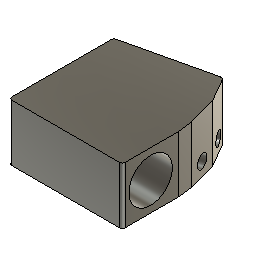
ornithopter (Autodesk Fusion 360 archive; units mm, degrees)
design "spar connector v2.0"
Autodesk Fusion 360 part; units mm, degrees
(part 1 of 2)
sketch "Sketch1" plane through (0, 0, 0) normal (0, 0, 1) x (1, 0, 0)
  line L0 (0, 0) -> (20, 0)
  line L1 (0, 0) -> (20, 0)
  line L2 (20, 0) -> (20, -5)
  line L3 (20, -5) -> (0, -5)
  line L4 (0, -5) -> (0, 0)
  line L5 (20, 0) -> (20, 5)
  line L6 (0, 0) -> (20, 0)
  line L7 (20, 0) -> (20, 5)
  line L8 (20, 5) -> (0, 5)
  line L9 (0, 5) -> (0, 0)
  line L10 (0, 5) -> (18.9894, 10.0882)
  line L11 (0, 5) -> (17.0254, 14.8296)
  line L12 (18.9894, 10.0882) -> (18.3195, 12.5882)
  line L13 (18.3195, 12.5882) -> (15.7313, 17.0711)
  line L14 (0, 5) -> (26.9466, 16.1616)
  line L15 (0, 5) -> (33.8519, 9.4567)
  line L16 (18.9894, 10.0882) -> (19.6593, 7.5882)
  line L17 (19.6593, 7.5882) -> (20, 5)
  line L18 (15.7313, 17.0711) -> (0, 5)
  line L19 (0, 5) -> (0, 13.4392)
  line L20 (0, 13.4392) -> (15.7313, 17.0711)
  dimension "d3" = 20
  dimension "d4" = 5
  dimension "d14" = 15
  dimension "d15" = 15
  dimension "d16" = 7.5
  dimension "d17" = 7.5
  dimension "d37" = 103
  dimension "d38" = 7.5
  constraint coincident L0.start L1.start
  constraint horizontal L0
  constraint horizontal L1
  constraint vertical L2
  constraint horizontal L3
  constraint vertical L4
  constraint perpendicular L1 L5
  constraint equal L2 L5
  constraint horizontal L6
  constraint vertical L7
  constraint horizontal L8
  constraint vertical L9
  constraint perpendicular L10 L12
  constraint perpendicular L11 L13
  constraint coincident L11.end L13
  constraint coincident L12.end L14
  constraint coincident L15 L16.end
  constraint perpendicular L10 L16
  constraint perpendicular L15 L17
  constraint perpendicular L8 L19
  measures "d3" distance of L0.start L0.end
  measures "d4" distance of L1 L3
  measures "d14" angle of L8 L10
  measures "d15" angle of L10 L11
  measures "d16" angle of L10 L14
  measures "d17" angle of L8 L15
  measures "d37" angle of L19 L20
  measures "d38" angle of L11 L18
extrude "Extrude1" add sketch "Sketch1" along normal blind 10
sketch "Sketch2" plane through (20, 0, 0) normal (1, 0, 0) x (0, 1, 0)
  line L0 (-5, 0) -> (5, 0)
  line L1 (5, 10) -> (-5, 10)
  line L2 (-5, 10) -> (-5, 0)
  line L3 (5, 0) -> (5, 10)
  point P0 (0, 5)
hole "Hole1" at (20, 0, 5) direction (-1, 0, 0) diameter 7.65 depth 20 tip angle 118
sketch "Sketch4" plane through (20.2394, 5.4231, 0) normal (0.965926, 0.258819, 0) x (-0.258819, 0.965926, 0)
  line L0 (2.2414, 0) -> (7.4178, 0)
  line L1 (7.4178, 0) -> (7.4178, 10)
  line L2 (7.4178, 10) -> (2.2414, 10)
  line L3 (2.2414, 10) -> (2.2414, 0)
  line L4 (2.2414, 2.35) -> (7.4178, 2.35)
  point P0 (4.8296, 2.35)
  dimension "d18" = 2.35
  constraint coincident L3 L4.start
  constraint coincident L1 L4.end
  constraint perpendicular L1 L4
  constraint midpoint L4 P0
  measures "d18" distance of L0 P0
sketch "Sketch5" plane through (19.1905, 11.0796, 0) normal (0.866025, 0.5, 0) x (-0.5, 0.866025, 0)
  line L0 (1.7419, 0) -> (6.9183, 0)
  line L1 (6.9183, 10) -> (1.7419, 10)
  line L2 (1.7419, 10) -> (1.7419, 0)
  line L3 (1.7419, 2.35) -> (7.3386, 2.35)
  line L4 (6.9183, 0) -> (6.9183, 10)
  point P0 (4.5403, 2.35)
  dimension "d19" = 2.35
  constraint coincident L2 L3.start
  constraint midpoint L3 P0
  measures "d19" distance of L0 L3
sketch "Sketch6" plane through (-2.9457, 12.7591, 0) normal (-0.224951, 0.97437, 0) x (-0.97437, -0.224951, 0)
  line L0 (-19.1683, 0) -> (-3.0232, 0)
  line L1 (-3.0232, 0) -> (-3.0232, 10)
  line L2 (-3.0232, 10) -> (-19.1683, 10)
  line L3 (-19.1683, 10) -> (-19.1683, 0)
  line L4 (-19.1683, 2.85) -> (-3.0232, 2.85)
  point P0 (-8.0232, 2.85)
  dimension "d43" = 2.85
  dimension "d47" = 5
  constraint coincident L3 L4.start
  constraint coincident L1 L4.end
  constraint perpendicular L1 L4
  constraint coincident L4 P0
  measures "d43" distance of L0 L4
  measures "d47" distance of L1 P0
hole "Hole4" at (4.8719, 14.564, 2.85) direction (0.224951, -0.97437, 0) diameter 3.35 depth 10 tip angle 118
hole "Hole2" at (18.9894, 10.0882, 2.35) direction (-0.965926, -0.258819, 0) diameter 2.35 depth 10 tip angle 118
hole "Hole3" at (16.9203, 15.0116, 2.35) direction (-0.866025, -0.5, 0) diameter 2.35 depth 10 tip angle 118
fillet "Fillet1" radius 0.5 1 edges at (15.7313, 17.0711, 5)
fillet "Fillet2" radius 0.5 1 edges at (20, -5, 5)
fillet "Fillet3" radius 0.5 1 edges at (0, 13.4392, 5)
fillet "Fillet4" radius 0.5 1 edges at (0, -5, 5)
mirror "Mirror1" [rolled back] mirror stitch tolerance 0.1
move_body "Move1" [rolled back]
equation "d18 = 5 mm - ( ( 7.65 * 0.5 ) * 1 mm ) + ( 2.35 * 0.5 ) * 1 mm"
equation "d19 = 5 mm - ( 7.65 * 0.5 ) * 1 mm + ( 2.35 * 0.5 ) * 1 mm"
equation "d37 = 180 deg - 77 deg"
equation "d43 = 5 mm - ( 7.65 * 0.5 ) * 1 mm + ( 3.35 * 0.5 ) * 1 mm"

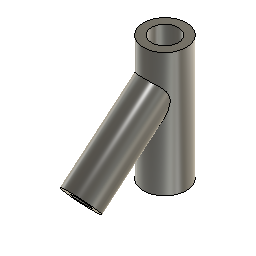
design "spar-to-screw connector"
Autodesk Fusion 360 part; units mm, degrees
sketch "Sketch1" plane through (0, 0, 0) normal (0, 0, 1) x (1, 0, 0)
  circle A0 centre (0, 0) radius 2.632
  circle A1 centre (0, 0) radius 1.632
  dimension "d1" = 3.2639
  dimension "d2" = 1
  constraint coincident A0.centre A1.centre
  constraint concentric A0 A1
  measures "d1" diameter of A1
  measures "d2" distance of A0 A1
extrude "Extrude1" add sketch "Sketch1" along normal blind 15.24 makes body 1
ref_plane "WorkPlane1" through (0, -2.632, 9.1335) normal (0, -1, 0) x (-1, 0, 0)
sketch "Sketch3" plane through (0, -2.632, 9.1335) normal (0, -1, 0) x (1, 0, 0)
  line L0 (-2.6886, 0) -> (2.6498, 0)
  constraint horizontal L0
ref_plane "WorkPlane2" through (-0.0194, -2.632, 9.1335) normal (0, 0.766044, 0.642788) x (1, 0, 0)
sketch "Sketch4" plane through (-0.0194, -2.632, 9.1335) normal (0, 0.766044, 0.642788) x (1, 0, 0)
  circle A0 centre (0, 0) radius 1.175
  circle A1 centre (0, 0) radius 2.175
  line L0 (0, 0) -> (-2.175, 0)
  line L1 (0, 0) -> (2.175, 0)
  dimension "d13" = 2.35
  dimension "d14" = 1
  constraint coincident A0.centre A1.centre
  constraint coincident A1 L0.end
  constraint horizontal L0
  constraint coincident A1 L1.end
  constraint parallel L0 L1
  measures "d13" diameter of A0
  measures "d14" distance of A0 A1
extrude "Extrude4" add sketch "Sketch4" along normal blind 3 separate body contours A0 A1 L0 L1 | A0 A1 L0 L1 makes body 2
extrude "Extrude6" add sketch "Sketch4" against normal blind 10 separate body contours A0 A1 L0 L1 | A0 A1 L0 L1 makes body 3
extrude "Extrude5" cut sketch "Sketch1" along normal blind 16 contours A1 bodies 2
extrude "Extrude7" cut sketch "Sketch1" along normal blind 16 contours A1 bodies 3
combine "Combine1" operation add target body 3 tool bodies 2 1

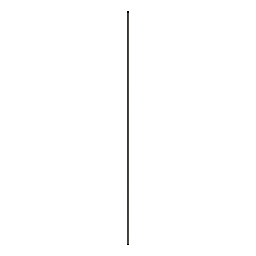
design "small spar medium"
Autodesk Fusion 360 part; units mm, degrees
sketch "Sketch1" plane through (0, 0, 0) normal (0, 0, 1) x (1, 0, 0)
  circle A0 centre (0, 0) radius 1
  dimension "d1" = 2
  constraint coincident A0.centre origin
  measures "d1" diameter of A0
extrude "Extrude1" add sketch "Sketch1" along normal blind 380

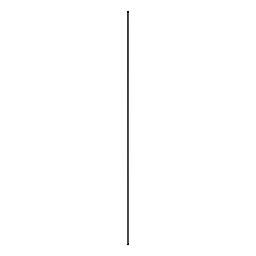
design "small spar long"
Autodesk Fusion 360 part; units mm, degrees
sketch "Sketch1" plane through (0, 0, 0) normal (0, 0, 1) x (1, 0, 0)
  circle A0 centre (0, 0) radius 1
  dimension "d1" = 2
  constraint coincident A0.centre origin
  measures "d1" diameter of A0
extrude "Extrude1" add sketch "Sketch1" along normal blind 423

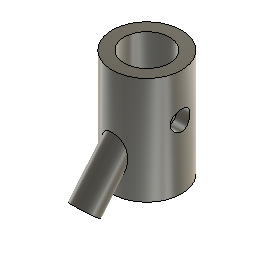
design "spar-to-spar connector large"
Autodesk Fusion 360 part; units mm, degrees
sketch "Sketch1" plane through (0, 0, 0) normal (0, 0, 1) x (1, 0, 0)
  circle A0 centre (0, 0) radius 5.75
  circle A1 centre (0, 0) radius 3.75
  dimension "d1" = 7.5
  dimension "d2" = 2
  constraint coincident A0.centre A1.centre
  constraint concentric A0 A1
  measures "d1" diameter of A1
  measures "d2" distance of A0 A1
extrude "Extrude1" add sketch "Sketch1" along normal blind 17.78 makes body 1
ref_plane "WorkPlane1" through (0, -5.75, 19.9539) normal (0, -1, 0) x (-1, 0, 0)
sketch "Sketch3" plane through (0, -5.75, 9.1335) normal (0, -1, 0) x (1, 0, 0)
  line L0 (-2.6886, 0) -> (2.6498, 0)
  constraint horizontal L0
ref_plane "WorkPlane2" through (-0.0194, -5.75, 9.1335) normal (0, 0.642788, 0.766044) x (1, 0, 0)
sketch "Sketch4" plane through (-0.0194, -3.9203, 7.5982) normal (0, 0.642788, 0.766044) x (1, 0, 0)
  circle A0 centre (0, 0) radius 1.175
  circle A1 centre (0, 0) radius 2.175
  line L0 (0, 0) -> (-2.175, 0)
  line L1 (0, 0) -> (2.175, 0)
  dimension "d13" = 2.35
  dimension "d14" = 1
  constraint coincident A0.centre A1.centre
  constraint coincident A1 L0.end
  constraint horizontal L0
  constraint coincident A1 L1.end
  constraint parallel L0 L1
  measures "d13" diameter of A0
  measures "d14" distance of A0 A1
extrude "Extrude4" add sketch "Sketch4" along normal blind 3 separate body contours A0 A1 L0 L1 | A0 A1 L0 L1 makes body 2
extrude "Extrude6" add sketch "Sketch4" against normal blind 10 separate body contours A0 A1 L0 L1 | A0 A1 L0 L1 makes body 3
extrude "Extrude5" cut sketch "Sketch1" along normal blind 16 contours A1 bodies 2
extrude "Extrude7" cut sketch "Sketch1" along normal blind 16 contours A1 bodies 3
combine "Combine1" operation add target body 3 tool bodies 2 1
ref_plane "WorkPlane3" through (5.75, 0, 13.4902) normal (1, 0, 0) x (0, -1, 0)
sketch "Sketch5" plane through (5.75, 0, 10.5576) normal (1, 0, 0) x (0, 1, 0)
  circle A0 centre (0, 0) radius 1.632
  dimension "d24" = 3.2639
  constraint coincident A0.centre origin
  measures "d24" diameter of A0
extrude "Extrude8" cut sketch "Sketch5" against normal blind 4 bodies 3

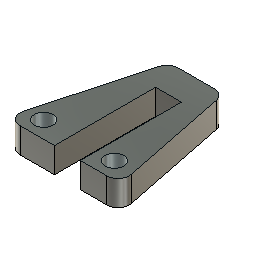
design "screw connector"
Autodesk Fusion 360 part; units mm, degrees
sketch "Sketch1" plane through (0, 0, 0) normal (0, 0, 1) x (1, 0, 0)
  line L0 (15.475, 10) -> (7.4034, 10)
  line L1 (8.375, 10) -> (12.975, 10)
  line L2 (12.975, 10) -> (12.975, 5)
  line L3 (12.975, 5) -> (8.375, 5)
  line L4 (8.375, 5) -> (8.375, 10)
  circle A0 centre (3.4375, -10) radius 1.651
  circle A1 centre (16.05, -10) radius 1.651
  line L5 (5.875, 10) -> (8.375, 10)
  line L6 (12.975, 10) -> (13.8399, 10)
  line L7 (5.4736, 8.5253) -> (0.3022, -10.4747)
  line L8 (2.232, -13) -> (17.693, -13)
  line L9 (19.6531, -10.6025) -> (15.8, 8.3975)
  arc A2 (7.4034, 10) -> (5.4736, 8.5253) centre (7.4034, 8) ccw
  arc A3 (15.8, 8.3975) -> (13.8399, 10) centre (13.8399, 8) ccw
  arc A4 (0.3022, -10.4747) -> (2.232, -13) centre (2.232, -11) ccw
  arc A5 (17.693, -13) -> (19.6531, -10.6025) centre (17.693, -11) ccw
  line L10 (8.375, 5) -> (8.375, -13)
  line L11 (12.975, 5) -> (12.975, -13)
  point P0 (0, 10)
  dimension "d9" = 4.6
  dimension "d11" = 3.302
  dimension "d21" = 20
  dimension "d22" = 20
  dimension "d23" = 2.5
  dimension "d24" = 2.5
  dimension "d25" = 3
  dimension "d26" = 2
  dimension "d27" = 2
  dimension "d28" = 2
  dimension "d29" = 2
  constraint horizontal L0
  constraint horizontal L1
  constraint vertical L2
  constraint horizontal L3
  constraint vertical L4
  constraint coincident L0 L1.start
  constraint equal A0 A1
  constraint coincident P0 L0
  constraint perpendicular L4 L5
  constraint parallel L5 L8
  constraint coincident L5.start L7
  constraint tangent L0 A2
  constraint tangent L7 A2
  constraint coincident L0.start L6
  constraint coincident L0.start L9
  constraint tangent L6 A3
  constraint tangent L9 A3
  constraint tangent L7 A4
  constraint tangent L8 A4
  constraint tangent L8 A5
  constraint tangent L9 A5
  constraint coincident L8 L10.end
  constraint perpendicular L8 L10
  constraint coincident L8 L11.end
  constraint perpendicular L8 L11
  measures "d9" distance of L2 L4
  measures "d11" diameter of A0
  measures "d21" distance of L0 A0.centre
  measures "d22" distance of L0 A1.centre
  measures "d23" distance of L1.start L5.start
  measures "d24" distance of L1.end L0.start
  measures "d25" distance of A0.centre L8
  measures "d26" radius of A2
  measures "d27" radius of A3
  measures "d28" radius of A4
  measures "d29" radius of A5
extrude "Extrude1" add sketch "Sketch1" along normal blind 4.5 contours L0 L2 L6 L8 L9 A3 A5 L11 | L0 L1 L2 L3 L4 | L0 L4 L5 L7 L8 A2 A4 L10
sketch "Sketch2" plane through (0, 0, 4.5) normal (0, 0, 1) x (-1, 0, 0)
  circle A0 centre (-3.4375, 10) radius 1.651
  circle A1 centre (-16.05, 10) radius 1.651
  line L0 (-8.375, -5) -> (-12.975, -5)
  line L1 (-12.975, -5) -> (-12.975, 13)
  line L2 (-12.975, 13) -> (-17.693, 13)
  arc A2 (-17.693, 13) -> (-19.6531, 10.6025) centre (-17.693, 11) ccw
  line L3 (-19.6531, 10.6025) -> (-15.8, -8.3975)
  arc A3 (-15.8, -8.3975) -> (-13.8399, -10) centre (-13.8399, -8) ccw
  line L4 (-13.8399, -10) -> (-7.4034, -10)
  arc A4 (-7.4034, -10) -> (-5.4736, -8.5253) centre (-7.4034, -8) ccw
  line L5 (-5.4736, -8.5253) -> (-0.3022, 10.4747)
  arc A5 (-0.3022, 10.4747) -> (-2.232, 13) centre (-2.232, 11) ccw
  line L6 (-2.232, 13) -> (-8.375, 13)
  line L7 (-8.375, 13) -> (-8.375, -5)

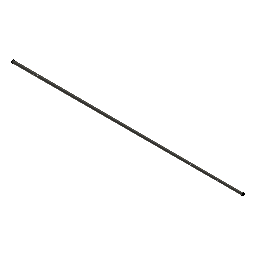
design "large spar"
Autodesk Fusion 360 part; units mm, degrees
sketch "Sketch1" plane through (0, 0, 0) normal (0, 0, 1) x (1, 0, 0)
  line L0 (0, 0) -> (825.5, 0)
  line L1 (825.5, 0) -> (825.5, 7.239)
  line L2 (825.5, 7.239) -> (0, 7.239)
  line L3 (0, 7.239) -> (0, 0)
  line L4 (825.5, 6.4135) -> (825.5, 7.239)
  line L5 (825.5, 1.4097) -> (825.5, 0)
  line L6 (825.5, 0.8255) -> (825.5, 0)
  line L7 (825.5, 6.4135) -> (825.5, 7.239)
  line L8 (825.5, 5.8293) -> (825.5, 6.4135)
  line L9 (825.5, 1.4097) -> (825.5, 0.8255)
  line L10 (0, 6.7183) -> (0, 7.239)
  line L11 (0, 0.5207) -> (0, 0)
  line L12 (0, 6.7183) -> (825.5, 5.8293)
  line L13 (825.5, 1.4097) -> (0, 0.5207)
  line L14 (0, 0) -> (825.5, 0.8255)
  line L15 (825.5, 6.4135) -> (0, 7.239)
  line L16 (0, 3.6195) -> (825.5, 3.6195)
  line L17 (600, 7.239) -> (600, 0)
  point P0 (825.5, 6.4135)
  point P1 (825.5, 5.8293)
  point P2 (825.5, 1.4097)
  point P3 (825.5, 0.8255)
  point P4 (0, 6.7183)
  point P5 (0, 0.5207)
  dimension "d1" = 7.239
  dimension "d2" = 825.5
  dimension "d3" = 5.588
  dimension "d4" = 4.4196
  dimension "d5" = 6.1976
  dimension "d7" = 600
  constraint horizontal L0
  constraint horizontal L2
  constraint vertical L3
  constraint coincident L0.start L3.end
  constraint coincident L1 P0
  constraint coincident L1 P2
  constraint coincident L1 P3
  constraint coincident P0 L4.start
  constraint coincident P2 L5.start
  constraint coincident P3 L6.start
  constraint equal L6 L7
  constraint coincident L1 P1
  constraint coincident P1 L8.start
  constraint equal L8 L9
  constraint coincident L3 P4
  constraint coincident L3 P5
  constraint coincident P4 L10.start
  constraint coincident P5 L11.start
  constraint equal L10 L11
  constraint midpoint L3 L16.start
  constraint midpoint L1 L16.end
  constraint coincident L2 L17.start
  constraint coincident L0 L17.end
  constraint perpendicular L0 L17
  measures "d1" distance of L0 L2
  measures "d2" distance of L1 L3
  measures "d3" distance of P0 P3
  measures "d4" distance of P1 P2
  measures "d5" distance of P4 P5
  measures "d7" distance of L3 L17
revolve "Revolve2" add sketch "Sketch1" angle 360 about axis through (0, 3.6195, 0) along (1, 0, 0) contours L3 L10 L12 L15 L17

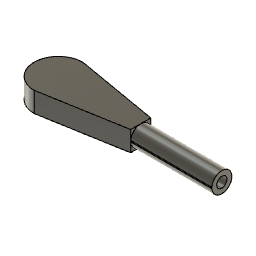
design "servo arm"
Autodesk Fusion 360 part; units mm, degrees
sketch "Sketch1" plane through (0, 0, 0) normal (0, 0, 1) x (1, 0, 0)
  line L0 (0, 0) -> (14.4, 0)
  line L1 (14.4, 0) -> (14.4, 15)
  line L2 (14.4, 15) -> (0, 15)
  line L3 (0, 15) -> (0, 0)
  circle A0 centre (0, 7.5) radius 7.5
  line L4 (0, 15) -> (14.4, 12.5)
  line L5 (0, 0) -> (14.4, 2.5)
  line L6 (14.4, 12.5) -> (25.3509, 10.5988)
  line L7 (14.4, 2.5) -> (25.3509, 4.4012)
  line L8 (25.3509, 4.4012) -> (25.3509, 10.5988)
  dimension "d1" = 15
  dimension "d2" = 14.4
  dimension "d3" = 10
  dimension "d4" = 6.1976
  constraint horizontal L0
  constraint vertical L1
  constraint horizontal L2
  constraint vertical L3
  constraint coincident L0.start L3.end
  constraint midpoint L3 A0.centre
  constraint coincident L2.end A0
  constraint coincident L1 L4.end
  constraint coincident L1 L5.end
  constraint equal L4 L5
  constraint parallel L4 L6
  constraint parallel L5 L7
  constraint coincident L7 L8.start
  constraint coincident L6 L8.end
  constraint perpendicular L2 L8
  constraint coincident L7.end L8.start
  constraint coincident L6.end L8.end
  measures "d1" distance of L0 L2
  measures "d2" distance of L1 L3
  measures "d3" distance of L4.end L5.end
  measures "d4" distance of L7.end L6.end
extrude "Extrude1" add sketch "Sketch1" along normal blind 6.1976 contours L3 A0 | L3 A0 L4 L5 | L1 A0 L4 L5 | L1 L6 L7 L8
sketch "Sketch2" plane through (25.3509, 0, 0) normal (1, 0, 0) x (0, 1, 0)
  line L0 (4.4012, 0) -> (10.5988, 0)
  line L1 (10.5988, 0) -> (10.5988, 6.1976)
  line L2 (10.5988, 6.1976) -> (4.4012, 6.1976)
  line L3 (4.4012, 6.1976) -> (4.4012, 0)
  circle A0 centre (7.4943, 3.0988) radius 3.0988
  circle A1 centre (7.4943, 3.0988) radius 1.5875
  dimension "d7" = 3.175
  constraint tangent L2 A0
  constraint tangent L0 A0
  constraint concentric A0 A1
  measures "d7" diameter of A1
extrude "Extrude2" add sketch "Sketch2" along normal blind 25 contours L3 A0 picked at (7.6808, 0.5158)

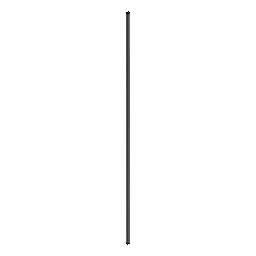
design "medium spar"
Autodesk Fusion 360 part; units mm, degrees
sketch "Sketch1" plane through (0, 0, 0) normal (0, 0, 1) x (1, 0, 0)
  circle A0 centre (0, 0) radius 1.5
  dimension "d1" = 3
  constraint coincident A0.centre origin
  measures "d1" diameter of A0
extrude "Extrude1" add sketch "Sketch1" along normal blind 240

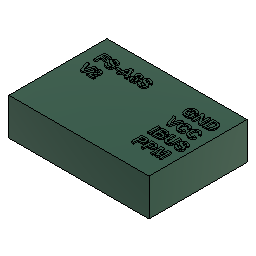
design "reciever"
Autodesk Fusion 360 part; units mm, degrees
sketch "Sketch1" plane through (0, 0, 0) normal (0, 0, 1) x (1, 0, 0)
  line L0 (0, 0) -> (20, 0)
  line L1 (20, 0) -> (20, 14)
  line L2 (20, 14) -> (0, 14)
  line L3 (0, 14) -> (0, 0)
  dimension "d1" = 20
  dimension "d2" = 14
  constraint horizontal L0
  constraint vertical L1
  constraint horizontal L2
  constraint vertical L3
  constraint coincident L0.start L3.end
  measures "d1" distance of L1 L3
  measures "d2" distance of L0 L2
extrude "Extrude1" add sketch "Sketch1" along normal blind 5.3
sketch "Sketch2" plane through (0, 0, 5.3) normal (0, 0, 1) x (-1, 0, 0)
  line L0 (0, -14) -> (0, 0)
  line L1 (0, 0) -> (-20, 0)
  line L2 (-20, 0) -> (-20, -14)
  line L3 (-20, -14) -> (0, -14)
  line L4 (-1.6357, -6.6523) -> (-11.9926, -6.6523) construction
  line L5 (-11.9926, -6.6523) -> (-11.9926, -11.8308) construction
  line L6 (-11.9926, -11.8308) -> (-1.6357, -11.8308) construction
  line L7 (-1.6357, -11.8308) -> (-1.6357, -6.6523) construction
  line L8 (-14.4693, -2.7122) -> (-20, -2.7122) construction
  line L9 (-20, -2.7122) -> (-20, -11.3805) construction
  line L10 (-20, -11.3805) -> (-14.4693, -11.3805) construction
  line L11 (-14.4693, -11.3805) -> (-14.4693, -2.7122) construction
  text T0 "FS-A8S\nV2" font "Arial" height 1.5 bold align left top in box 10.3569 x 5.1784 at (-1.6357, -6.6523) x (-1, 0) y (0, -1) spacing 1 kerned
  text T1 "GND\nVCC\nIBUS\nPPM" font "Arial" height 1.5 bold align left top in box 5.5307 x 8.6683 at (-14.4693, -2.7122) x (-1, 0) y (0, -1) spacing 1 kerned
  constraint coincident L2
emboss "Emboss1" depth 0.2 profiles "Sketch2" section 1 text T1 T0 onto face at (6.6667, 9.3333, 5.3)

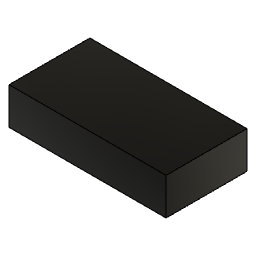
design "battery"
Autodesk Fusion 360 part; units mm, degrees
sketch "Sketch1" plane through (0, 0, 0) normal (0, 0, 1) x (1, 0, 0)
  line L0 (0, 0) -> (68, 0)
  line L1 (68, 0) -> (68, 35)
  line L2 (68, 35) -> (0, 35)
  line L3 (0, 35) -> (0, 0)
  dimension "d1" = 68
  dimension "d2" = 35
  constraint horizontal L0
  constraint vertical L1
  constraint horizontal L2
  constraint vertical L3
  constraint coincident L0.start L3.end
  measures "d1" distance of L1 L3
  measures "d2" distance of L0 L2
extrude "Extrude1" add sketch "Sketch1" along normal blind 16

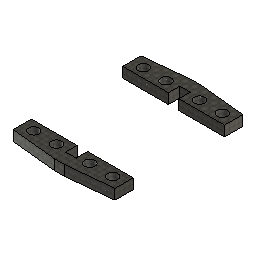
design "servo mount"
Autodesk Fusion 360 part; units mm, degrees
sketch "Sketch1" plane through (0, 0, 0) normal (0, 0, 1) x (1, 0, 0)
  line L0 (0, 0) -> (44.6, 0)
  line L1 (44.6, 0) -> (44.6, 60)
  line L2 (44.6, 60) -> (0, 60)
  line L3 (0, 60) -> (0, 0)
  line L4 (20, 0) -> (36.7004, 0)
  line L5 (0, 0) -> (44.6, 0)
  line L6 (44.6, 0) -> (44.6, 10)
  line L7 (44.6, 10) -> (0, 10)
  line L8 (0, 10) -> (0, 0)
  line L9 (44.6, 60) -> (0, 60)
  line L10 (0, 60) -> (0, 50)
  line L11 (0, 50) -> (44.6, 50)
  line L12 (44.6, 50) -> (44.6, 60)
  line L13 (24.6, 0) -> (44.6, 2)
  line L14 (0, 2) -> (20, 0)
  line L15 (0, 58) -> (20, 60)
  line L16 (24.6, 60) -> (44.6, 58)
  line L17 (20, 50) -> (24.6, 50)
  line L18 (24.6, 50) -> (24.6, 60)
  line L19 (24.6, 60) -> (20, 60)
  line L20 (20, 60) -> (20, 50)
  line L21 (20, 55) -> (24.6, 55)
  line L22 (24.6, 55) -> (24.6, 50)
  line L23 (24.6, 50) -> (20, 50)
  line L24 (20, 50) -> (20, 55)
  line L25 (20, 0) -> (24.6, 0)
  line L26 (24.6, 0) -> (24.6, 10)
  line L27 (24.6, 10) -> (20, 10)
  line L28 (20, 10) -> (20, 0)
  line L29 (20, 10) -> (24.6, 10)
  line L30 (24.6, 10) -> (24.6, 5)
  line L31 (24.6, 5) -> (20, 5)
  line L32 (20, 5) -> (20, 10)
  dimension "d2" = 60
  dimension "d17" = 10
  dimension "d18" = 10
  dimension "d37" = 2
  dimension "d43" = 20
  dimension "d44" = 2
  dimension "d45" = 20
  dimension "d46" = 20
  dimension "d47" = 20
  dimension "d48" = 2
  dimension "d49" = 2
  dimension "d59" = 5
  dimension "d60" = 5
  dimension "d61" = 4.6
  dimension "d62" = 4.6
  constraint horizontal L0
  constraint vertical L1
  constraint horizontal L2
  constraint vertical L3
  constraint coincident L0.start L3.end
  constraint horizontal L4
  constraint coincident L0 L4.start
  constraint horizontal L5
  constraint vertical L6
  constraint horizontal L7
  constraint vertical L8
  constraint coincident L1 L6.end
  constraint horizontal L9
  constraint vertical L10
  constraint horizontal L11
  constraint vertical L12
  constraint coincident L3 L10.end
  constraint coincident L1 L13.end
  constraint coincident L0 L13.start
  constraint coincident L8 L14.start
  constraint coincident L3 L15.start
  constraint coincident L2 L15.end
  constraint coincident L2 L16.start
  constraint coincident L1 L16.end
  constraint horizontal L17
  constraint vertical L18
  constraint horizontal L19
  constraint vertical L20
  constraint coincident L11 L17.start
  constraint horizontal L21
  constraint vertical L22
  constraint horizontal L23
  constraint vertical L24
  constraint coincident L20 L21.start
  constraint horizontal L25
  constraint vertical L26
  constraint horizontal L27
  constraint vertical L28
  constraint coincident L7 L26.end
  constraint horizontal L29
  constraint vertical L30
  constraint horizontal L31
  constraint vertical L32
  constraint coincident L26 L30.end
  constraint coincident L4.start L14.end
  measures "d2" distance of L0 L2
  measures "d17" distance of L5 L7
  measures "d18" distance of L2 L11
  measures "d37" distance of L5 L13.end
  measures "d43" distance of L1 L13.start
  measures "d44" distance of L0.start L14.start
  measures "d45" distance of L0.start L4.start
  measures "d46" distance of L3 L15.end
  measures "d47" distance of L1 L16.start
  measures "d48" distance of L1.end L16.end
  measures "d49" distance of L2.end L15.start
  measures "d59" distance of L17 L21
  measures "d60" distance of L7 L31
  measures "d61" distance of L26 L28
  measures "d62" distance of L22 L24
extrude "Extrude4" add sketch "Sketch1" along normal blind 4.5 contours L0 L4 L5 L25 L26 L28 L31 | L3 L7 L8 L14 L28 L32 | L1 L6 L7 L13 L26 L30 | L3 L10 L11 L15 L20 L24 | L1 L11 L12 L16 L18 L22 | L2 L9 L18 L19 L20 L21 makes body 1 at (6.6667, 54.3333, 0) makes body 2 at (6.6667, 5.6667, 0)
sketch "Sketch3" plane through (0, 0, 4.5) normal (0, 0, 1) x (-1, 0, 0)
  line L0 (-44.6, -50) -> (-44.6, -58)
  line L1 (0, -58) -> (0, -50)
  line L2 (0, -50) -> (-20, -50)
  line L3 (0, -54) -> (-44.6, -54)
  line L4 (-24.6, -60) -> (-20, -60)
  line L5 (-44.6, -58) -> (-24.6, -60)
  line L6 (-20, -60) -> (0, -58)
  line L7 (-20, -50) -> (-20, -55)
  line L8 (-20, -55) -> (-24.6, -55)
  line L9 (-24.6, -55) -> (-24.6, -50)
  line L10 (-24.6, -50) -> (-44.6, -50)
  point P0 (-5, -54)
  point P1 (-15, -54)
  point P2 (-39.6, -54)
  point P3 (-29.6, -54)
  dimension "d24" = 5
  dimension "d25" = 10
  dimension "d26" = 5
  dimension "d27" = 10
  dimension "d50" = 6
  constraint coincident P0 L3
  constraint coincident P1 L3
  constraint coincident P3 L3
  constraint coincident P2 L3
  constraint coincident L0 L3.end
  measures "d24" distance of L1 P0
  measures "d25" distance of P0 P1
  measures "d26" distance of P2 L3.end
  measures "d27" distance of P2 P3
  measures "d50" distance of L3 L4
hole "Hole1" at (5, 54, 4.5) at (15, 54, 4.5) at (29.6, 54, 4.5) at (39.6, 54, 4.5) direction (0, 0, -1) diameter 4.5 depth 20 tip angle 118 bodies 1
sketch "Sketch4" plane through (0, 0, 4.5) normal (0, 0, 1) x (-1, 0, 0)
  line L0 (0, -10) -> (0, -2)
  line L1 (-44.6, -2) -> (-44.6, -10)
  line L2 (-20, -10) -> (0, -10)
  line L3 (0, -6) -> (-44.6, -6)
  line L4 (-24.6, 0) -> (-44.6, -2)
  line L5 (-20, 0) -> (-24.6, 0)
  line L6 (0, -2) -> (-20, 0)
  line L7 (-20, -5) -> (-20, -10)
  line L8 (-44.6, -10) -> (-24.6, -10)
  line L9 (-24.6, -10) -> (-24.6, -5)
  line L10 (-24.6, -5) -> (-20, -5)
  point P0 (-5, -6)
  point P1 (-15, -6)
  point P2 (-29.6, -6)
  point P3 (-39.6, -6)
  dimension "d28" = 5
  dimension "d29" = 10
  dimension "d30" = 5
  dimension "d31" = 10
  dimension "d40" = 6
  constraint coincident L3 P0
  constraint coincident L3 P1
  constraint coincident L3 P2
  constraint coincident L3 P3
  constraint coincident L1 L3.end
  measures "d28" distance of L0 P0
  measures "d29" distance of P0 P1
  measures "d30" distance of L3.end P3
  measures "d31" distance of P2 P3
  measures "d40" distance of L3 L4.start
hole "Hole2" at (5, 6, 4.5) at (15, 6, 4.5) at (29.6, 6, 4.5) at (39.6, 6, 4.5) direction (0, 0, -1) diameter 4.5 depth 20 tip angle 118 bodies 2

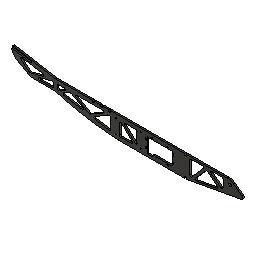
design "frame v2.0"
Autodesk Fusion 360 part; units mm, degrees
sketch "Sketch2" plane through (0, 0, 0) normal (0, 1, 0) x (1, 0, 0)
  line L0 (0, 0) -> (650, 0)
  line L1 (650, 0) -> (650, -200)
  line L2 (650, -200) -> (0, -200)
  line L3 (0, -200) -> (0, 0)
  line L4 (0, -81.4313) -> (0, -60)
  line L5 (54, -30) -> (0, -60)
  line L6 (54, -30) -> (121.5, -29.9038)
  line L7 (121.5, -29.9038) -> (121.4776, -14.1987)
  line L8 (121.5, -29.9038) -> (121.5429, -60)
  line L9 (121.5429, -60) -> (610.012, -60)
  line L10 (610.012, -60) -> (650, -30)
  line L11 (650, -30) -> (486, 0)
  line L12 (486, 0) -> (297, 0)
  line L13 (297, 0) -> (121.4776, -14.1987)
  line L14 (0, -81.4313) -> (121.5429, -60)
  point P0 (650, -679.9029)
  point P1 (201.3394, 90.956)
  point P2 (486, 0)
  point P3 (-7419.8633, 0)
  point P4 (0, -60)
  point P5 (0, -81.4313)
  point P6 (121.5429, -60)
  point P7 (54, -30)
  point P8 (121.5, -29.9038)
  point P9 (121.4776, -14.1987)
  point P10 (297, 0)
  point P11 (650, -30)
  point P12 (610.012, -60)
  dimension "d5" = 650
  dimension "d6" = 200
  dimension "d30" = 60
  dimension "d32" = 30
  dimension "d33" = 54
  dimension "d34" = 121.5
  dimension "d36" = 60
  dimension "d37" = 297
  dimension "d38" = 486
  dimension "d39" = 30
  dimension "d40" = 60
  dimension "d80" = 170
  constraint horizontal L0
  constraint vertical L1
  constraint horizontal L2
  constraint vertical L3
  constraint coincident L0.start L3.end
  constraint coincident L1 P0
  constraint coincident L0 P2
  constraint coincident L0 P3
  constraint coincident L3 P4
  constraint coincident L3 P5
  constraint coincident L0 P10
  constraint coincident L1 P11
  constraint coincident P5 L4.start
  constraint coincident P4 L4.end
  constraint coincident P7 L5.start
  constraint coincident P8 L6.end
  constraint coincident P9 L7.end
  constraint perpendicular L6 L7
  constraint coincident P6 L8.end
  constraint parallel L7 L8
  constraint coincident P12 L9.end
  constraint coincident P11 L10.end
  constraint coincident P2 L11.end
  constraint coincident P10 L12.end
  measures "d5" distance of L1 L3
  measures "d6" distance of L0 L2
  measures "d30" distance of L0 P4
  measures "d32" distance of L0 P7
  measures "d33" distance of L3 P7
  measures "d34" distance of L3 P8
  measures "d36" distance of L0 P6
  measures "d37" distance of L0.start P10
  measures "d38" distance of L3 P2
  measures "d39" distance of L0 P11
  measures "d40" distance of L0 P12
  measures "d80" angle of L9 L14
extrude "Extrude3" add sketch "Sketch2" along normal blind 4.5 contours L0 L7 L8 L9 L10 L11 L12 L13 | L3 L4 L5 L6 L8 L14
sketch "Sketch4" plane through (0, 0, 0) normal (0, -1, 0) x (1, 0, 0)
  line L0 (0, 81.4313) -> (0, 60)
  line L1 (0, 60) -> (54, 30)
  line L2 (54, 30) -> (121.5, 29.9038)
  line L3 (121.5, 29.9038) -> (121.4776, 14.1987)
  line L4 (121.4776, 14.1987) -> (297, 0)
  line L5 (297, 0) -> (486, 0)
  line L6 (486, 0) -> (650, 30)
  line L7 (650, 30) -> (610.012, 60)
  line L8 (610.012, 60) -> (121.5429, 60)
  line L9 (486, 0) -> (481.4, 0)
  line L10 (481.4, 0) -> (481.4, 60)
  line L11 (481.4, 60) -> (486, 60)
  line L12 (486, 60) -> (486, 0)
  line L13 (481.4, 60) -> (486, 60)
  line L14 (486, 60) -> (486, 55)
  line L15 (486, 55) -> (481.4, 55)
  line L16 (481.4, 55) -> (481.4, 60)
  line L17 (481.4, 0) -> (486, 0)
  line L18 (486, 0) -> (486, 5)
  line L19 (486, 5) -> (481.4, 5)
  line L20 (481.4, 5) -> (481.4, 0)
  line L21 (121.5429, 60) -> (0, 81.4313)
  dimension "d57" = 4.6
  dimension "d58" = 5
  constraint horizontal L9
  constraint vertical L10
  constraint horizontal L11
  constraint vertical L12
  constraint coincident L8 L10.end
  constraint coincident L5.end L6.start
  constraint horizontal L13
  constraint vertical L14
  constraint horizontal L15
  constraint vertical L16
  constraint coincident L12 L14.end
  constraint horizontal L17
  constraint vertical L18
  constraint horizontal L19
  constraint vertical L20
  constraint equal L16 L20
  measures "d57" distance of L10 L12
  measures "d58" distance of L5 L19.end
extrude "Extrude5" cut sketch "Sketch4" against normal blind 5 contours L8 L10 L11 L12 L13 L14 L15 L16 | L5 L9 L10 L12 L17 L18 L19 L20
fillet "Fillet16" radius 730 1 edges at (121.4776, 2.25, 14.1987)
fillet "Fillet17" radius 5 1 edges at (650, 2.25, 30)
fillet "Fillet18" radius 30 1 edges at (610.012, 2.25, 60)
fillet "Fillet19" radius 30 1 edges at (54, 2.25, 30)
fillet "Fillet20" radius 30 1 edges at (0, 2.25, 60)
fillet "Fillet22" radius 5 1 edges at (0, 2.25, 81.4313)
sketch "Sketch21" plane through (0, 0, 0) normal (0, -1, 0) x (1, 0, 0)
  arc A0 (5.9649, 80.3795) -> (0.116, 75.0161) centre (5.0967, 75.4555) ccw
  arc A1 (0.116, 75.0161) -> (15.4307, 51.4274) centre (30, 77.6521) ccw
  line L0 (15.4307, 51.4274) -> (47.2244, 33.7642)
  arc A2 (47.2244, 33.7642) -> (61.751, 29.989) centre (61.7937, 59.9889) ccw
  line L1 (61.751, 29.989) -> (121.5, 29.9038)
  arc A3 (121.5, 29.9038) -> (270.1218, 2.1743) centre (328.9822, 729.7974) ccw
  line L2 (270.1218, 2.1743) -> (297, 0)
  line L3 (297, 0) -> (481.4, 0)
  line L4 (481.4, 0) -> (481.4, 5)
  line L5 (481.4, 5) -> (486, 5)
  line L6 (486, 5) -> (486, 0)
  line L7 (486, 0) -> (638.7541, 27.9428)
  arc A4 (638.7541, 27.9428) -> (640.855, 36.8608) centre (637.8544, 32.8612) ccw
  line L8 (640.855, 36.8608) -> (618.013, 53.9974)
  arc A5 (618.013, 53.9974) -> (600.0096, 60) centre (600.0096, 30) ccw
  line L9 (600.0096, 60) -> (486, 60)
  line L10 (486, 60) -> (486, 55)
  line L11 (486, 55) -> (481.4, 55)
  line L12 (481.4, 55) -> (481.4, 60)
  line L13 (481.4, 60) -> (121.5429, 60)
  line L14 (121.5429, 60) -> (5.9649, 80.3795)
  line L15 (121.5429, 60) -> (5.9649, 80.3795)
  line L16 (5.9649, 80.3795) -> (4.6452, 72.895)
  line L17 (4.6452, 72.895) -> (120.2232, 52.5155)
  line L18 (120.2232, 52.5155) -> (121.5429, 60)
  line L19 (121.022, 57.0456) -> (5.444, 77.4251)
  line L20 (4.6452, 72.895) -> (5.444, 77.4251)
  line L21 (5.444, 77.4251) -> (-21.9849, 82.2615)
  line L22 (-21.9849, 82.2615) -> (-22.7836, 77.7314)
  line L23 (-22.7836, 77.7314) -> (4.6452, 72.895)
  line L24 (55.444, 68.6087) -> (54.6452, 64.0786)
  dimension "d201" = 50
  dimension "d213" = 4.6
  dimension "d215" = 3
  constraint perpendicular L15 L16
  constraint parallel L15 L17
  constraint parallel L16 L18
  constraint coincident A0.start L14.end
  constraint tangent A0 L15
  constraint coincident L13.end L14.start
  constraint perpendicular L20 L21
  constraint parallel L20 L22
  constraint parallel L21 L23
  constraint coincident L19 L24.start
  constraint coincident L17 L24.end
  constraint perpendicular L17 L24
  constraint parallel L19 L21
  constraint parallel L15 L19
  measures "d201" horizontal distance of L16.end L24.end
  measures "d213" distance of L21 L23
  measures "d215" distance of L15 L19
extrude "Extrude13" cut sketch "Sketch21" against normal blind 10 contours A0 A1 L16 L20 L21 L23 | L16 L17 L19 L20 L24
sketch "Sketch7" plane through (0, 0, 0) normal (0, -1, 0) x (1, 0, 0)
  arc A0 (0.2658, 73.6672) -> (15.4307, 51.4274) centre (30, 77.6521) ccw
  line L0 (15.4307, 51.4274) -> (47.2244, 33.7642)
  arc A1 (47.2244, 33.7642) -> (61.751, 29.989) centre (61.7937, 59.9889) ccw
  line L1 (61.751, 29.989) -> (121.5, 29.9038)
  arc A2 (121.5, 29.9038) -> (270.1218, 2.1743) centre (328.9822, 729.7974) ccw
  line L2 (270.1218, 2.1743) -> (297, 0)
  line L3 (297, 0) -> (481.4, 0)
  line L4 (481.4, 0) -> (481.4, 5)
  line L5 (481.4, 5) -> (486, 5)
  line L6 (486, 5) -> (486, 0)
  line L7 (486, 0) -> (638.7541, 27.9428)
  arc A3 (638.7541, 27.9428) -> (640.855, 36.8608) centre (637.8544, 32.8612) ccw
  line L8 (640.855, 36.8608) -> (618.013, 53.9974)
  arc A4 (618.013, 53.9974) -> (600.0096, 60) centre (600.0096, 30) ccw
  line L9 (600.0096, 60) -> (486, 60)
  line L10 (486, 60) -> (486, 55)
  line L11 (486, 55) -> (481.4, 55)
  line L12 (481.4, 55) -> (481.4, 60)
  line L13 (378.4, 48) -> (445.4, 48)
  line L14 (446.4, 48) -> (446.4, 12)
  line L15 (445.4, 12) -> (378.4, 12)
  line L16 (377.4, 12) -> (377.4, 47)
  line L17 (377.4, 48) -> (377.4, 60)
  line L18 (377.4, 12) -> (377.4, 0)
  line L19 (481.4, 60) -> (121.5429, 60)
  line L20 (121.5429, 60) -> (5.9649, 80.3795)
  arc A5 (5.9649, 80.3795) -> (0.931, 78.2208) centre (5.0967, 75.4555) ccw
  line L21 (377.4, 51) -> (446.4, 51)
  line L22 (446.4, 51) -> (446.4, 53)
  line L23 (446.4, 53) -> (377.4, 53)
  line L24 (377.4, 53) -> (377.4, 51)
  line L25 (377.4, 7) -> (446.3768, 7)
  line L26 (446.3768, 7) -> (446.3768, 9)
  line L27 (446.3768, 9) -> (377.4, 9)
  line L28 (377.4, 9) -> (377.4, 7)
  line L29 (377.4, 48) -> (374.4, 48)
  line L30 (374.4, 48) -> (374.4, 12)
  line L31 (374.4, 12) -> (377.4, 12)
  line L32 (377.4, 12) -> (377.4, 48)
  line L33 (374.4, 12) -> (372.4, 12)
  line L34 (372.4, 12) -> (372.4, 48)
  line L35 (372.4, 48) -> (374.4, 48)
  line L36 (374.4, 48) -> (374.4, 12)
  line L37 (446.4, 48) -> (449.4, 48)
  line L38 (449.4, 48) -> (449.4, 12)
  line L39 (449.4, 12) -> (446.4, 12)
  line L40 (446.4, 13) -> (446.4, 47)
  line L41 (449.4, 12) -> (451.4, 12)
  line L42 (451.4, 12) -> (451.4, 48)
  line L43 (451.4, 48) -> (449.4, 48)
  line L44 (449.4, 48) -> (449.4, 12)
  line L45 (377.4, 51) -> (377.4, 48)
  line L46 (377.4, 9) -> (377.4, 12)
  line L47 (387.4, 53) -> (392.4, 53)
  line L48 (392.4, 53) -> (392.4, 51)
  line L49 (392.4, 51) -> (387.4, 51)
  line L50 (387.4, 51) -> (387.4, 53)
  line L51 (431.4, 53) -> (436.4, 53)
  line L52 (436.4, 53) -> (436.4, 51)
  line L53 (436.4, 51) -> (431.4, 51)
  line L54 (431.4, 51) -> (431.4, 53)
  line L55 (387.4, 9) -> (392.4, 9)
  line L56 (392.4, 9) -> (392.4, 7)
  line L57 (392.4, 7) -> (387.4, 7)
  line L58 (387.4, 7) -> (387.4, 9)
  line L59 (431.3768, 9) -> (436.3768, 9)
  line L60 (436.3768, 9) -> (436.3768, 7)
  line L61 (436.3768, 7) -> (431.3768, 7)
  line L62 (431.3768, 7) -> (431.3768, 9)
  line L63 (449.4, 43) -> (451.4, 43)
  line L64 (451.4, 43) -> (451.4, 38)
  line L65 (451.4, 38) -> (449.4, 38)
  line L66 (449.4, 38) -> (449.4, 43)
  line L67 (449.4, 22) -> (451.4, 22)
  line L68 (451.4, 22) -> (451.4, 17)
  line L69 (451.4, 17) -> (449.4, 17)
  line L70 (449.4, 17) -> (449.4, 22)
  line L71 (372.4, 43) -> (374.4, 43)
  line L72 (374.4, 43) -> (374.4, 38)
  line L73 (374.4, 38) -> (372.4, 38)
  line L74 (372.4, 38) -> (372.4, 43)
  line L75 (372.4, 22) -> (374.4, 22)
  line L76 (374.4, 22) -> (374.4, 17)
  line L77 (374.4, 17) -> (372.4, 17)
  line L78 (372.4, 17) -> (372.4, 22)
  line L79 (377.4, 53) -> (387.4, 53)
  line L80 (436.4, 53) -> (446.4, 53)
  line L81 (446.3768, 9) -> (436.3768, 9)
  line L82 (387.4, 9) -> (377.4, 9)
  line L83 (446.4, 51) -> (446.4, 48)
  line L84 (451.4, 17) -> (451.4, 22)
  line L85 (372.4, 43) -> (372.4, 48)
  line L86 (372.4, 17) -> (372.4, 12)
  line L87 (451.4, 12) -> (451.4, 17)
  line L88 (451.4, 43) -> (451.4, 48)
  line L89 (377.4, 12) -> (372.4, 12)
  line L90 (372.4, 12) -> (377.4, 12)
  line L91 (377.4, 12) -> (377.4, 7)
  line L92 (377.4, 7) -> (372.4, 7)
  line L93 (372.4, 7) -> (372.4, 12)
  arc A6 (378.4, 48) -> (377.4, 47) centre (378.4, 47) ccw
  arc A7 (446.4, 47) -> (445.4, 48) centre (445.4, 47) ccw
  arc A8 (445.4, 12) -> (446.4, 13) centre (445.4, 13) ccw
  line L94 (378.4, 12) -> (377.4, 12)
  line L95 (392.4, 7) -> (392.4, 12)
  line L96 (377.4, 7) -> (387.4, 7)
  line L97 (387.4, 7) -> (387.4, 9)
  line L98 (387.4, 9) -> (377.4, 9)
  line L99 (377.4, 9) -> (377.4, 7)
  line L100 (54.6452, 64.0786) -> (0.2658, 73.6672)
  line L101 (0.931, 78.2208) -> (55.444, 68.6087)
  line L102 (55.444, 68.6087) -> (54.6452, 64.0786)
  dimension "d75" = 69
  dimension "d76" = 36
  dimension "d79" = 35
  dimension "d88" = 3
  dimension "d89" = 2
  dimension "d90" = 10
  dimension "d91" = 5
  dimension "d92" = 5
  dimension "d192" = 1
  dimension "d194" = 1
  dimension "d195" = 1
  constraint horizontal L13
  constraint vertical L14
  constraint horizontal L15
  constraint vertical L16
  constraint coincident L3 L18.end
  constraint perpendicular L3 L18
  constraint equal L17 L18
  constraint horizontal L21
  constraint vertical L22
  constraint horizontal L23
  constraint vertical L24
  constraint coincident L17 L21.start
  constraint horizontal L25
  constraint vertical L26
  constraint horizontal L27
  constraint vertical L28
  constraint coincident L18 L25.start
  constraint horizontal L29
  constraint vertical L30
  constraint horizontal L31
  constraint vertical L32
  constraint horizontal L33
  constraint vertical L34
  constraint horizontal L35
  constraint vertical L36
  constraint horizontal L37
  constraint vertical L38
  constraint horizontal L39
  constraint vertical L40
  constraint horizontal L41
  constraint vertical L42
  constraint horizontal L43
  constraint vertical L44
  constraint perpendicular L13 L45
  constraint equal L45 L46
  constraint equal L31 L45
  constraint equal L39 L46
  constraint equal L28 L35
  constraint equal L28 L41
  constraint equal L24 L28
  constraint coincident L29.end L30.start
  constraint coincident L37 L38.start
  constraint horizontal L47
  constraint vertical L48
  constraint horizontal L49
  constraint vertical L50
  constraint coincident L21 L48.end
  constraint coincident L23 L47.start
  constraint horizontal L51
  constraint vertical L52
  constraint horizontal L53
  constraint vertical L54
  constraint coincident L21 L52.end
  constraint coincident L23 L51.start
  constraint horizontal L55
  constraint vertical L56
  constraint horizontal L57
  constraint vertical L58
  constraint coincident L25 L56.end
  constraint coincident L27 L55.start
  constraint horizontal L59
  constraint vertical L60
  constraint horizontal L61
  constraint vertical L62
  constraint coincident L25 L60.end
  constraint coincident L27 L59.start
  constraint horizontal L63
  constraint vertical L64
  constraint horizontal L65
  constraint vertical L66
  constraint coincident L42 L64.end
  constraint coincident L38 L63.start
  constraint horizontal L67
  constraint vertical L68
  constraint horizontal L69
  constraint vertical L70
  constraint coincident L42 L68.end
  constraint coincident L38 L67.start
  constraint horizontal L71
  constraint vertical L72
  constraint horizontal L73
  constraint vertical L74
  constraint coincident L30 L72.end
  constraint coincident L34 L71.start
  constraint horizontal L75
  constraint vertical L76
  constraint horizontal L77
  constraint vertical L78
  constraint coincident L36 L76.end
  constraint coincident L34 L75.start
  constraint equal L79 L80
  constraint equal L80 L81
  constraint equal L81 L82
  constraint perpendicular L13 L83
  constraint equal L49 L53
  constraint equal L49 L72
  constraint equal L74 L78
  constraint equal L55 L78
  constraint equal L57 L61
  constraint equal L61 L66
  constraint equal L64 L68
  constraint equal L87 L88
  constraint equal L86 L87
  constraint equal L85 L86
  constraint coincident L16.start L18.start
  constraint coincident L14.end L39.end
  constraint coincident L17.end L19
  constraint horizontal L89
  constraint horizontal L90
  constraint vertical L91
  constraint horizontal L92
  constraint vertical L93
  constraint coincident L17.start L13
  constraint tangent L16 A6
  constraint tangent L13 A6
  constraint coincident L16.start L15
  constraint coincident L14.start L13
  constraint tangent L13 A7
  constraint tangent L40 A7
  constraint coincident L14.end L40
  constraint coincident L14.end L15
  constraint tangent L40 A8
  constraint tangent L15 A8
  constraint coincident L15 L95.end
  constraint perpendicular L15 L95
  constraint horizontal L96
  constraint vertical L97
  constraint horizontal L98
  constraint vertical L99
  measures "d75" distance of L14 L16
  measures "d76" distance of L13 L15
  measures "d79" distance of L11.end L14
  measures "d88" distance of L13 L21
  measures "d89" distance of L21 L23
  measures "d90" distance of L23.end L47.start
  measures "d91" distance of L47.start L47.end
  measures "d92" distance of L34.end L71.start
  measures "d192" radius of A6
  measures "d194" radius of A7
  measures "d195" radius of A8
extrude "Extrude12" cut sketch "Sketch7" against normal blind 10 contours L18 L25 L27 L28 L58 L82 L91 L96 L97 L98 L99 | L21 L23 L47 L48 L49 L50 | L15 L18 L27 L46 L55 L82 L91 L94 L95 L98 | L25 L27 L55 L56 L57 L58 L95 L97 | L13 L14 L15 L16 L32 L40 A6 A7 A8 L94 | L21 L23 L51 L52 L53 L54 | L25 L27 L59 L60 L61 L62 | L30 L34 L36 L75 L76 L77 L78 | L30 L34 L36 L71 L72 L73 L74 | L38 L42 L44 L63 L64 L65 L66 | L38 L42 L44 L67 L68 L69 L70 L84
sketch "Sketch11" plane through (0, 0, 0) normal (0, -1, 0) x (1, 0, 0)
  arc A0 (5.9649, 80.3795) -> (0.931, 78.2208) centre (5.0967, 75.4555) ccw
  arc A1 (0.2658, 73.6672) -> (15.4307, 51.4274) centre (30, 77.6521) ccw
  line L0 (15.4307, 51.4274) -> (47.2244, 33.7642)
  arc A2 (47.2244, 33.7642) -> (61.751, 29.989) centre (61.7937, 59.9889) ccw
  line L1 (61.751, 29.989) -> (121.5, 29.9038)
  arc A3 (121.5, 29.9038) -> (270.1218, 2.1743) centre (328.9822, 729.7974) ccw
  line L2 (270.1218, 2.1743) -> (297, 0)
  line L3 (297, 0) -> (481.4, 0)
  line L4 (481.4, 0) -> (481.4, 5)
  line L5 (481.4, 5) -> (486, 5)
  line L6 (486, 5) -> (486, 0)
  line L7 (486, 0) -> (638.7541, 27.9428)
  arc A4 (638.7541, 27.9428) -> (640.855, 36.8608) centre (637.8544, 32.8612) ccw
  line L8 (640.855, 36.8608) -> (618.013, 53.9974)
  arc A5 (618.013, 53.9974) -> (600.0096, 60) centre (600.0096, 30) ccw
  line L9 (600.0096, 60) -> (486, 60)
  line L10 (486, 60) -> (486, 55)
  line L11 (486, 55) -> (481.4, 55)
  line L12 (481.4, 55) -> (481.4, 60)
  line L13 (481.4, 60) -> (121.5429, 60)
  line L14 (121.5429, 60) -> (5.9649, 80.3795)
  line L15 (290.245, 49.685) -> (358.825, 49.685)
  line L16 (358.825, 49.685) -> (358.825, 10.315)
  line L17 (358.825, 10.315) -> (290.245, 10.315)
  line L18 (290.245, 10.315) -> (290.245, 49.685)
  line L19 (290.245, 49.685) -> (290.245, 60)
  line L20 (358.825, 10.315) -> (358.825, 0)
  line L21 (436.3768, 9) -> (436.3768, 7)
  line L22 (436.3768, 7) -> (431.3768, 7)
  line L23 (431.3768, 7) -> (431.3768, 9)
  line L24 (431.3768, 9) -> (436.3768, 9)
  line L25 (392.4, 53) -> (392.4, 51)
  line L26 (392.4, 51) -> (387.4, 51)
  line L27 (387.4, 51) -> (387.4, 53)
  line L28 (387.4, 53) -> (392.4, 53)
  line L29 (436.4, 53) -> (436.4, 51)
  line L30 (436.4, 51) -> (431.4, 51)
  line L31 (431.4, 51) -> (431.4, 53)
  line L32 (431.4, 53) -> (436.4, 53)
  line L33 (451.4, 22) -> (451.4, 17)
  line L34 (451.4, 17) -> (449.4, 17)
  line L35 (449.4, 17) -> (449.4, 22)
  line L36 (449.4, 22) -> (451.4, 22)
  line L37 (374.4, 22) -> (374.4, 17)
  line L38 (374.4, 17) -> (372.4, 17)
  line L39 (372.4, 17) -> (372.4, 22)
  line L40 (372.4, 22) -> (374.4, 22)
  line L41 (392.4, 7) -> (377.4, 7)
  line L42 (377.4, 7) -> (377.4, 47)
  arc A6 (378.4, 48) -> (377.4, 47) centre (378.4, 47) ccw
  line L43 (378.4, 48) -> (445.4, 48)
  arc A7 (446.4, 47) -> (445.4, 48) centre (445.4, 47) ccw
  line L44 (446.4, 47) -> (446.4, 13)
  arc A8 (445.4, 12) -> (446.4, 13) centre (445.4, 13) ccw
  line L45 (445.4, 12) -> (392.4, 12)
  line L46 (392.4, 12) -> (392.4, 7)
  line L47 (374.4, 43) -> (374.4, 38)
  line L48 (374.4, 38) -> (372.4, 38)
  line L49 (372.4, 38) -> (372.4, 43)
  line L50 (372.4, 43) -> (374.4, 43)
  line L51 (451.4, 43) -> (451.4, 38)
  line L52 (451.4, 38) -> (449.4, 38)
  line L53 (449.4, 38) -> (449.4, 43)
  line L54 (449.4, 43) -> (451.4, 43)
  line L55 (54.6452, 64.0786) -> (0.2658, 73.6672)
  line L56 (0.931, 78.2208) -> (55.444, 68.6087)
  line L57 (55.444, 68.6087) -> (54.6452, 64.0786)
  dimension "d95" = 68.58
  dimension "d96" = 39.37
  constraint horizontal L15
  constraint vertical L16
  constraint horizontal L17
  constraint vertical L18
  constraint coincident L13 L19.end
  constraint perpendicular L13 L19
  constraint coincident L3 L20.end
  constraint perpendicular L3 L20
  constraint equal L19 L20
  measures "d95" distance of L16 L18
  measures "d96" distance of L15 L17
hole "Hole1" at (358.825, 0, 49.685) at (290.245, 0, 49.685) at (290.245, 0, 10.315) at (358.825, 0, 10.315) direction (0, 1, 0) diameter 3.2639 depth 20 tip angle 118
hole "Hole2" at (608.0806, 0, 47.3768) direction (0, 1, 0) diameter 8 depth 20 tip angle 118